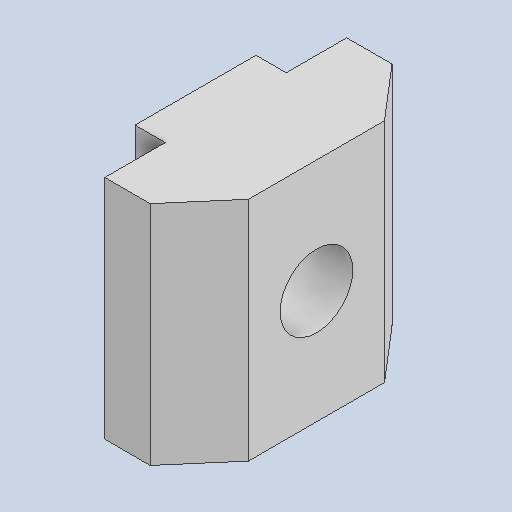
# Autodesk Inventor part: drazkaVel
Saved by Autodesk Inventor 2025 (Build 290162000, 162)
## iProperties
Created: 2025-09-03
Part Number: drazkaVel
Material: Generic
Document SubType Name: Modeling
Designer: Pravoslav
Density: 1 g/cm^3
Appearance: Default
Author: Pravoslav
Autodesk Inventor part; units mm, degrees
ref_plane "YZ Plane" through (0, 0, 0) normal (1, 0, 0) x (0, 1, 0)
ref_plane "XZ Plane" through (0, 0, 0) normal (0, 1, 0) x (-1, 0, 0)
ref_plane "XY Plane" through (0, 0, 0) normal (0, 0, 1) x (1, 0, 0)
sketch "Sketch1" plane through (0, 0, 0) normal (0, 1, 0) x (-1, 0, 0)
  line L0 (3, 8) -> (-3, 8)
  line L1 (-3, 8) -> (-3, -8)
  line L2 (-3, -8) -> (3, -8)
  line L3 (3, -8) -> (3, 8)
  line L4 (3, 8) -> (-3, -8) construction
  line L5 (-3, 8) -> (3, -8) construction
  line L6 (5, 4) -> (1, 4)
  line L7 (1, 4) -> (1, -4)
  line L8 (1, -4) -> (5, -4)
  line L9 (5, -4) -> (5, 4)
  line L10 (5, 4) -> (1, -4) construction
  line L11 (1, 4) -> (5, -4) construction
  line L12 (0, 8) -> (-3, 4.5)
  line L13 (-3, -4.5) -> (0, -8)
  point P0 (0, 0)
  point P1 (3, 0)
  point P2 (-3, 0)
  point P3 (3, 4)
  point P4 (3, -4)
  dimension "d0" = 6
  dimension "d1" = 16
  dimension "d2" = 4
  dimension "d3" = 8
  dimension "d4" = 3
  dimension "d5" = 3
  dimension "d6" = 9
  dimension "d7" = 4.5
  constraints: 28 end point, 8 midpoint, 4 parallel, 2 horizontal, 2 perpendicular, 2 point on line
  measures "d0" distance of L2.end L1.end
  measures "d1" distance of L1.end L0.end
  measures "d2" distance of L8.end L7.end
  measures "d3" distance of L7.end L6.end
  measures "d4" distance from line of L3 L12.start
  measures "d5" distance of L13.end L2.end
  measures "d6" distance of L13.start L12.end
  measures "d7" distance of point (-3, 0) L12.end
extrude "Extrusion1" add sketch "Sketch1" along normal blind 15 contours L3 L6 L7 L8 L2 L13 L1 L12 L0 | L6 L9 L8 L3 | L3 L8 L7 L6
sketch "Sketch2" plane through (-5, 0, -4) normal (-1, 0, 0) x (0, 0, 1)
  circle A0 centre (4, 7.5) radius 2.4
  line L0 (0, 0) -> (8, 0) projected
  line L1 (8, 0) -> (8, 15) projected
  point P0 (4, 0)
  dimension "d10" = 4.8
  dimension "d11" = 7.5
  dimension "d12" = 4
  constraints: 1 centre point
  measures "d10" diameter of A0
  measures "d11" distance from line of L0 A0.centre
  measures "d12" distance from line of L1 A0.centre
extrude "Extrusion2" cut sketch "Sketch2" against normal through all
body "Solid1"
